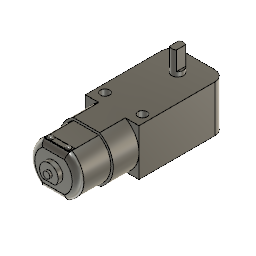
MotorReductor v1 (Autodesk Fusion 360 design; units mm, degrees)
Autodesk Fusion 360 part; units mm, degrees
note: some values were not read from the file. Set by a fixed rule: which sketch regions a step uses.
sketch "Boceto1" plane through (0, 0, 0) normal (0, 0, 1) x (1, 0, 0)
  line L0 (-11.5, 32) -> (11.5, 32) construction
  line L1 (11.5, 32) -> (11.5, -32) construction
  line L2 (11.5, -32) -> (-11.5, -32) construction
  line L3 (-11.5, -32) -> (-11.5, 32) construction
  line L4 (0, 1.75) -> (0, 22.5) construction
  line L5 (1.75, 0) -> (22.5, 0) construction
  line L6 (-7, 32) -> (7, 32)
  line L7 (11.5, 27.5) -> (11.5, -5)
  line L8 (11.5, -5) -> (-11.5, -5)
  line L9 (-11.5, -5) -> (-11.5, 27.5)
  arc A0 (-7, 32) -> (-11.5, 27.5) centre (-7, 27.5) ccw
  arc A1 (11.5, 27.5) -> (7, 32) centre (7, 27.5) ccw
  circle A2 centre (0, 23) radius 2.5
  circle A3 centre (-8, 0) radius 1.924
  circle A4 centre (8, 0) radius 1.924
  line L10 (-1.5, 25) -> (-1.5, 21)
  line L11 (1.5, 25) -> (1.5, 21)
  point P0 (11.5, 32)
  dimension "d1" = 64
  dimension "d2" = 23
  dimension "d3" = 23
  dimension "d4" = 37
  dimension "d5" = 4.5
  dimension "d6" = 5
  dimension "d7" = 9
  constraint horizontal L0
  constraint vertical L1
  constraint horizontal L2
  constraint vertical L3
  constraint symmetric L1 L3 L4
  constraint symmetric L0 L2 L5
  constraint horizontal L6
  constraint vertical L7
  constraint horizontal L8
  constraint vertical L9
  constraint coincident L0.start L9
  constraint coincident L0.start L6
  constraint tangent L9 A0
  constraint tangent L6 A0
  constraint coincident P0 L6
  constraint coincident P0 L7
  constraint tangent L6 A1
  constraint tangent L7 A1
  constraint equal A0 A1
  constraint coincident L4 A2.centre
  constraint coincident L5 A3.centre
  constraint coincident L5 A4.centre
  constraint equal A3 A4
  constraint coincident A2 L10.start
  constraint coincident A2 L10.end
  constraint vertical L10
  constraint coincident A2 L11.start
  constraint coincident A2 L11.end
  constraint parallel L4 L11
  measures "d1" distance of P0 L1.end
  measures "d2" distance of L1.end L2.end
  measures "d3" distance of L0.start P0
  measures "d4" distance of L0.start L8.end
  measures "d5" radius of A0
  measures "d6" diameter of A2
  measures "d7" distance of L6 A2.centre
extrude "Extruir1" add sketch "Boceto1" along normal mid plane 24 contours A2 L11 | A2 L10 makes body 1 at (-1.6831, 24.8485, 4) makes body 2 at (1.6831, 24.8485, -4)
extrude "Extruir2" add sketch "Boceto1" along normal mid plane 40 contours A2 L10 L11 bodies 1 2
extrude "Extruir3" add sketch "Boceto1" along normal mid plane 20 bodies 1
sketch "Boceto2" plane through (0, -5, 0) normal (0, -1, 0) x (1, 0, 0)
  line L0 (11.5, -10) -> (11.5, 10)
  line L1 (11.5, 10) -> (-11.5, 10)
  line L2 (-11.5, 10) -> (-11.5, -10)
  line L3 (-11.5, -10) -> (11.5, -10)
  circle A0 centre (0, 0) radius 11.5
  point P0 (11.5, 0)
  constraint coincident A0.centre origin
  constraint coincident A0 P0
extrude "Extruir4" add sketch "Boceto2" along normal blind 11 contours L1 L3 A0 bodies 1
sketch "Boceto3" plane through (0, -16, 0) normal (0, -1, 0) x (1, 0, 0)
  arc A0 (5.6789, -10) -> (5.6789, 10) centre (0, 0) ccw
  line L0 (5.6789, 10) -> (-5.6789, 10)
  arc A1 (-5.6789, 10) -> (-5.6789, -10) centre (0, 0) ccw
  line L1 (-5.6789, -10) -> (5.6789, -10)
  arc A2 (5.4083, -9) -> (5.4083, 9) centre (0, 0) ccw
  line L2 (5.4083, 9) -> (-5.4083, 9)
  arc A3 (-5.4083, 9) -> (-5.4083, -9) centre (0, 0) ccw
  line L3 (-5.4083, -9) -> (5.4083, -9)
  dimension "d16" = -1
extrude "Extruir5" add sketch "Boceto3" along normal blind 14 contours A2 L2 A3 L3 bodies 1
fillet "Empalme1" radius 2.5 4 edges at (10.5, -30, 0) (0, -30, 9) (-10.5, -30, 0) (0, -30, -9) on bodies 1
sketch "Boceto4" plane through (0, 0, 9) normal (0, 0, 1) x (-1, 0, 0)
  line L0 (5.4083, 27.5) -> (-5.4083, 27.5)
  line L1 (-5.4083, 27.5) -> (-5.4083, 16)
  line L2 (-5.4083, 16) -> (5.4083, 16)
  line L3 (5.4083, 16) -> (5.4083, 27.5)
  circle A0 centre (3.7528, 27.5) radius 1.036
  line L4 (0, -2.5) -> (0, -20)
  circle A1 centre (-3.7528, 27.5) radius 1.036
  line L5 (5.4083, 26.2478) -> (-5.3244, 26.2478)
  line L6 (-5.3244, 26.2478) -> (-5.3244, 28.6878)
  line L7 (-5.3244, 28.6878) -> (5.4083, 28.6878)
  line L8 (5.4083, 28.6878) -> (5.4083, 26.2478)
  spline S0 degree 3 poles (-4.6637, 30) (-4.6645, 30) (-4.6653, 30) (-4.7232, 29.9995) (-4.7792, 29.98) (-4.8872, 29.9035) (-4.9389, 29.8468) (-5.0755, 29.6384) (-5.153, 29.4485) (-5.279, 28.9815) (-5.3272, 28.7124) (-5.392, 28.1252) (-5.4083, 27.8144) (-5.4083, 27.5) knots -0.402189 -0.402189 -0.402189 -0.402189 -0.401397 -0.401397 -0.34552 -0.34552 -0.289946 -0.289946 -0.190291 -0.190291 -0.094312 -0.094312 0 0 0 0
  constraint coincident L0 A0.centre
  constraint symmetric A0 L4 A1
  constraint horizontal L5
  constraint vertical L6
  constraint horizontal L7
  constraint vertical L8
  constraint coincident L6.end S0
  constraint coincident L3 L5.start
revolve "Revolución1" add sketch "Boceto4" angle 360 about axis through (-5.4083, -27.5, 9) along (1, 0, 0) contours L0 A0 | L0 A1 picked at (3.9255, 28.0987) picked at (-3.9513, 28.1434) bodies 1
extrude "Extruir6" add sketch "Boceto1" along normal mid plane 2 contours A3 | A4 bodies 1
extrude "Extruir7" add sketch "Boceto4" along normal mid plane 0.2 contours L0 L3 A0 A1 L5 L6 L8 | L0 A0 A1 L6 L7 L8 bodies 1
sketch "Boceto5" plane through (0, -30, 0) normal (0, -1, 0) x (1, 0, 0)
  arc A0 (-4.6637, 6.5) -> (-4.6637, -6.5) centre (0, 0) ccw
  line L0 (-4.6637, -6.5) -> (4.6637, -6.5)
  arc A1 (4.6637, -6.5) -> (4.6637, 6.5) centre (0, 0) ccw
  line L1 (4.6637, 6.5) -> (-4.6637, 6.5)
  circle A2 centre (0, 0) radius 4
  circle A3 centre (0, 0) radius 1.4113
  line L2 (-3, -3) -> (3, -3)
  constraint coincident A0.centre A1.centre
  constraint horizontal L2
extrude "Extruir8" add sketch "Boceto5" along normal blind 3 separate body contours A3 makes body 3
extrude "Extruir9" add sketch "Boceto5" along normal blind 2 contours A2 L2 picked at (0.0352, -2.4691) bodies 1 3
sketch "Boceto6" plane through (0, 0, 0) normal (0, 0, 1) x (1, 0, 0)
  line L0 (1.8951, 32) -> (-2.1049, 32)
  line L1 (-2.1049, 32) -> (-2.1049, 36.6031)
  line L2 (-2.1049, 36.6031) -> (1.8951, 36.6031)
  line L3 (1.8951, 36.6031) -> (1.8951, 32)
  line L4 (7, 32) -> (-7, 32)
  circle A0 centre (-0.1049, 34.3016) radius 1.1353
  dimension "d30" = 4
  constraint horizontal L0
  constraint vertical L1
  constraint horizontal L2
  constraint vertical L3
  constraint coincident L0.start L4
  measures "d30" distance of L0.start L0.end
extrude "Extruir10" add sketch "Boceto6" along normal mid plane 4 separate body makes body 4
